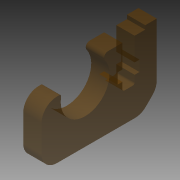
# Autodesk Inventor part: acrylic x bushing bracket
Saved by Autodesk Inventor 2014 SP1 (Build 180222100, 222)
## iProperties
Created: 2014-10-12
Part Number: acrylic x bushing bracket
Material: Polycarbonate, Smoke
Document SubType Name: Modeling
Designer: Mon
Density: 1.2 g/cm^3
Appearance: Polycarbonate - Smoked
Author: Mon
Autodesk Inventor part; units mm, degrees
ref_plane "YZ Plane" through (0, 0, 0) normal (1, 0, 0) x (0, 1, 0)
ref_plane "XZ Plane" through (0, 0, 0) normal (0, 1, 0) x (-1, 0, 0)
ref_plane "XY Plane" through (0, 0, 0) normal (0, 0, 1) x (1, 0, 0)
sketch "Sketch1" plane through (0, 0, 0) normal (1, 0, 0) x (0, 1, 0)
  line L0 (28.7426, 2.9397) -> (27.0858, 1.2829)
  arc A0 (24.2573, 0.1113) -> (27.0858, 1.2829) centre (24.2573, 4.1113) ccw
  line L1 (24.2573, 0.1113) -> (3.9142, 0.1113)
  arc A1 (-0.0858, 4.1113) -> (3.9142, 0.1113) centre (3.9142, 4.1113) ccw
  line L2 (-0.0858, 4.1113) -> (-0.0858, 11.1113)
  arc A2 (3.9142, 15.1113) -> (-0.0858, 11.1113) centre (3.9142, 11.1113) ccw
  line L3 (3.9142, 15.1113) -> (4.5315, 15.1113)
  arc A3 (28.7426, 2.9397) -> (29.9142, 5.7681) centre (25.9142, 5.7681) ccw
  arc A4 (5.023, 14.5191) -> (4.5315, 15.1113) centre (4.5315, 14.6113) ccw
  arc A5 (5.023, 14.5191) -> (16.3827, 17.1069) centre (11.2642, 13.3488) ccw
  arc A6 (17.1887, 18.6988) -> (16.3827, 17.1069) centre (17.1887, 17.6988) ccw
  line L4 (17.1887, 18.6988) -> (20.9642, 18.6988)
  line L5 (20.9642, 18.6988) -> (20.9642, 12.6988)
  line L6 (20.9642, 12.6988) -> (19.7042, 12.6988)
  line L7 (19.7042, 12.6988) -> (19.7042, 9.8988)
  line L8 (19.7042, 9.8988) -> (20.9642, 9.8988)
  line L9 (20.9642, 9.8988) -> (20.9642, 8.1988)
  arc A7 (20.9642, 8.1988) -> (21.4642, 7.6988) centre (21.4642, 8.1988) ccw
  line L10 (21.4642, 7.6988) -> (23.6642, 7.6988)
  arc A8 (23.6642, 7.6988) -> (24.1642, 8.1988) centre (23.6642, 8.1988) ccw
  line L11 (24.1642, 8.1988) -> (24.1642, 9.8988)
  line L12 (24.1642, 9.8988) -> (25.4242, 9.8988)
  line L13 (25.4242, 9.8988) -> (25.4242, 12.6988)
  line L14 (25.4242, 12.6988) -> (24.1642, 12.6988)
  line L15 (24.1642, 12.6988) -> (24.1642, 18.6988)
  line L16 (24.1642, 18.6988) -> (26.9142, 18.6988)
  line L17 (26.9142, 18.6988) -> (26.9142, 19.6988)
  line L18 (26.9142, 19.6988) -> (29.9142, 19.6988)
  line L19 (29.9142, 19.6988) -> (29.9142, 5.7681)
  point P0 (0, 0)
  constraints: 40 end point, 18 point on circle, 9 centre point
extrude "Extrusion1" add sketch "Sketch1" along normal blind 4.7625
body "Solid1"
